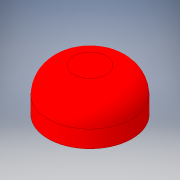
# Autodesk Inventor part: M211LC01W-led
Saved by Autodesk Inventor 2019 (Build 230136000, 136)
## iProperties
Created: 2022-08-22
Part Number: M211LC01W-led
Material: Generic
Catalog Web Link: www.cadenas.de
Description: M2100 Series LED Tipped Actuators - led-
Vendor: NKKSWITCHES
Document SubType Name: Modeling
Designer: psAdmin
Manufacturer: NKKSWITCHES
Mass: 0.00533918 g
Surface Area: 0.168484 cm^2
Volume: 0.00533918 cm^3
Density: 1 g/cm^3
Appearance: PSOLRGB-255-0-0
Category: PARTsolutions
Company: NKKSWITCHES
Title: M211LC01W-led
Author: Cadenas PARTsolutions
PSOL_IDENT_0: {$CADENAS_DATA/23d-libs/nkkswitches/toggle/m2100/parts/m2100_led.prj},223 {VTYP=3D},{NB=M211LC01W-le
PSOL_IDENT_1: d},{LINA=M211LC01W-led},{NN=M2100 Series LED Tipped Actuators - led},{DATE=02.08.2022 07:27:13},{GEO
PSOL_IDENT_2: MDATE=09.04.2009 00:00:00},{VERSION=},{LINEID=10},{WBVAR=PLS,LCAT,LEDCLR,CMRT,TMT},{WBNUMERIC=}  {NB=
PSOL_IDENT_3: M211LC01W-led},{LINA=M211LC01W-led},{KT=DUMMY},{PN=M211LC01W},{SRS=M21},{PLS=1},{LCAT=L},{LCAT1= 'L'
PSOL_IDENT_4: ,'L - Isolated (Toggle)','T','T - Synchronous (Toggle)','R','R - Isolated (Rocker)','N','N - Synchro
PSOL_IDENT_5: nous (Rocker)','P','P - Isolated (Paddle)','J','J - Synchronous (Paddle)' },{LEDCLR=C},{LEDCLRALG=1.
PSOL_IDENT_6: 00,0.00,0.00,0.00},{CMRT=W},{TMT=01},{TMT1= '01','01 - Solder Lug with Threaded Bushing','02','02 -
PSOL_IDENT_7: Quick Connect with Threaded Bushing','03','03 - Straight PC with Threaded Bushing' }
NB: M211LC01W-led
NN: M2100 Series LED Tipped Actuators - led
NBSYN: $PN.-led
LINA: M211LC01W-led
CATALOG: NKK Switches
PN: M211LC01W
SRS: M21
PLS: 1 - SPDT
LCAT: L - Isolated (Toggle)
LEDCLR: C - Red
CMRT: W - Silver; Rated 6A @ 125V AC
TMT: 01 - Solder Lug with Threaded Bushing
SUPPLIER: NKKSWITCHES
ARTICLENO: M211LC01W-led
BOMINFO: M211LC01W-led
CREATOR: CADENAS GmbH
Autodesk Inventor part; units mm, degrees
sketch "Sketch_1" plane through (0, 0, 0) normal (0, 0, 1) x (1, 0, 0)
  line L0 (0, 0) -> (0, 1.27)
  line L1 (0, 1.27) -> (0.4826, 1.27)
  arc A0 (1.2446, 0.508) -> (0.4826, 1.27) centre (0.4826, 0.508) ccw
  line L2 (1.2446, 0.508) -> (1.2446, 0)
  line L3 (1.2446, 0) -> (0, 0)
  line L4 (0, 0) -> (0, 1.27)
  constraints: 10 end point, 2 point on circle, 1 centre point
revolve "Revolution1" add sketch "Sketch_1" angle 360 about axis through (0, 0, 0) along (0, -1, 0)
ref_plane "full_led_to_act_XY" through (0, 0, 0) normal (0, -1, 0) x (1, 0, 0)
ref_plane "full_led_to_act_YZ" through (0, 0, 0) normal (1, 0, 0) x (0, 0, 1)
ref_plane "full_led_to_act_ZX" through (0, 0, 0) normal (0, 0, 1) x (0, -1, 0)
body "Solid1"
